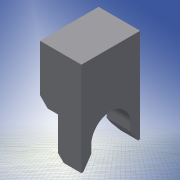
# Autodesk Inventor part: _WT_Aufnahme_Antriebseinheit6
Saved by Autodesk Inventor 2019 (Build 230136000, 136)
## iProperties
Created: 2025-05-01
Part Number: _WT_Aufnahme_Antriebseinheit6
Material: Generisch
Document SubType Name: Modeling
Designer: RP
Density: 1 g/cm^3
Appearance: Vorgabe
Author: RP
Autodesk Inventor part; units mm, degrees
ref_plane "YZ Plane" through (0, 0, 0) normal (1, 0, 0) x (0, 1, 0)
ref_plane "XZ Plane" through (0, 0, 0) normal (0, 1, 0) x (-1, 0, 0)
ref_plane "XY Plane" through (0, 0, 0) normal (0, 0, 1) x (1, 0, 0)
sketch "Skizze1" plane through (0, 0, 0) normal (0, 0, 1) x (1, 0, 0)
  line L0 (24.8274, -43.9228) -> (24.8274, -19.9228)
  line L1 (24.8274, -19.9228) -> (46.0274, -19.9228)
  line L2 (46.0274, -19.9228) -> (46.0274, -67.9228)
  line L3 (34.0274, -47.9228) -> (28.8274, -47.9228)
  line L4 (28.8274, -47.9228) -> (24.8274, -43.9228)
  line L5 (34.0274, -47.9228) -> (34.0274, -67.9228)
  line L6 (34.0274, -67.9228) -> (46.0274, -67.9228)
  point P0 (0, 0)
  dimension "d0" = 45
  dimension "d1" = 4
  dimension "d2" = 21.2
  dimension "d7" = 28
  dimension "d8" = 20
  dimension "d9" = 12
  constraints: 14 end point, 4 perpendicular, 2 vertical
  measures "d0" angle of L4 L0
  measures "d1" horizontal distance of L3.end L0.start
  measures "d2" distance of L0.end L1.end
  measures "d7" distance between parallel lines of L1 L3
  measures "d8" distance of L3.start L5.end
  measures "d9" distance of L5.end L2.end
extrude "Extrusion1" add sketch "Skizze1" along normal mid plane 30
sketch "Skizze2" plane through (46.0274, -67.9228, 15) normal (1, 0, 0) x (0, 0, -1)
  line L0 (5.0357, 14) -> (5.0357, 5)
  line L1 (5.0357, 5) -> (1.5346, 0)
  line L2 (1.5346, 0) -> (28.4654, 0)
  line L3 (0, 0) -> (30, 0) projected
  line L4 (28.4654, 0) -> (24.9643, 5)
  line L5 (24.9643, 5) -> (24.9643, 14)
  line L6 (24.9643, 14) -> (5.0357, 14) construction
  line L7 (15, -13.5846) -> (15, 81.5074) projected
  arc A0 (24.9643, 14) -> (18.9643, 20) centre (18.9643, 14) ccw
  line L8 (18.9643, 20) -> (11.0357, 20)
  arc A1 (11.0357, 20) -> (5.0357, 14) centre (11.0357, 14) ccw
  point P0 (15, 67.9228)
  dimension "d19" = 5
  dimension "d21" = 6
  dimension "d22" = 20
  dimension "d23" = 35
  constraints: 14 end point, 4 point on circle, 4 tangent, 2 centre point, 2 horizontal, 1 perpendicular, 1 point on line, 1 vertical, 2 other
  measures "d19" distance from line of L0.end L2
  measures "d21" radius of A1
  measures "d22" distance between parallel lines of L8 L2
  measures "d23" angle of L0 L1
extrude "Extrusion2" cut sketch "Skizze2" against normal through all
chamfer "Fase1" distance 3 angle 45 2 edges at (34.0274, -67.9228, -14.2327) (34.0274, -67.9228, 14.2327)
